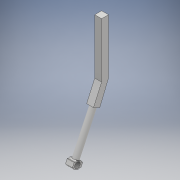
# Autodesk Inventor part: Fingers IPT
Saved by Autodesk Inventor 2017 (Build 210142000, 142)
## iProperties
Created: 2019-11-11
Part Number: Fingers IPT
Material: Generic
Document SubType Name: Modeling
Designer: kenli
Density: 1 g/cm^3
Appearance: Default
Author: kenli
Autodesk Inventor part; units mm, degrees
ref_plane "YZ Plane" through (0, 0, 0) normal (1, 0, 0) x (0, 1, 0)
ref_plane "XZ Plane" through (0, 0, 0) normal (0, 1, 0) x (-1, 0, 0)
ref_plane "XY Plane" through (0, 0, 0) normal (0, 0, 1) x (1, 0, 0)
sketch "Sketch1" plane through (0, 0, 0) normal (1, 0, 0) x (0, 1, 0)
  line L0 (3.4615, 28.4615) -> (-1.5385, 28.4615)
  line L1 (-1.5385, 28.4615) -> (-1.5385, -11.5385)
  line L2 (-1.5385, -11.5385) -> (3.4615, -11.5385)
  line L3 (3.4615, -11.5385) -> (3.4615, 28.4615)
  line L4 (3.4615, -11.5385) -> (-2.6923, -26.4744)
  line L5 (-2.8588, -26.8784) -> (-2.8558, -26.8796)
  line L6 (-2.8558, -26.8796) -> (-2.6923, -26.4744)
  line L7 (-2.8558, -26.8796) -> (-7.4503, -24.7123)
  line L8 (-7.4503, -24.7123) -> (-1.5385, -11.5385)
  point P0 (0, 0)
  dimension "d0" = 5
  dimension "d1" = 5.08
  dimension "d21" = 40
  constraints: 18 end point, 2 parallel, 2 perpendicular, 1 horizontal, 1 point on line
  measures "d0" distance between parallel lines of L1 L3
  measures "d1" distance of L5.end L7.end
  measures "d21" distance of L2.end L0.start
extrude "Extrusion1" add sketch "Sketch1" along normal blind 5
sketch "Sketch2" plane through (5, -2.8558, -26.8796) normal (0, -0.426635, -0.9044239) x (-1, 0, 0)
  circle A0 centre (2.5, -2.5) radius 2.0828
  line L0 (5, -5.08) -> (5, 0) projected
  line L1 (5, 0) -> (0, 0) projected
  point P0 (5, -8.885)
  dimension "d4" = 4.1656
  dimension "d5" = 2.5
  dimension "d6" = 2.5
  constraints: 1 centre point
  measures "d4" diameter of A0
  measures "d5" distance from line of A0.centre L0
  measures "d6" distance from line of A0.centre L1
extrude "Extrusion2" add sketch "Sketch2" along normal blind 30
sketch "Sketch7" plane through (2.5, -17.9159, -52.9458) normal (0, -0.426635, -0.9044239) x (-1, 0, 0)
  line L0 (2.5, -2.58) -> (-2.5, -2.58) projected
  line L1 (-2.5, 2.2849) -> (2.5, 2.2849)
  line L2 (2.5, 2.2849) -> (2.5, -2.58)
  line L3 (2.5, -2.58) -> (-2.5, -2.58)
  line L4 (-2.5, -2.58) -> (-2.5, 2.2849)
  point P0 (2.5, -6.385)
  constraints: 8 end point, 2 parallel, 1 horizontal, 1 perpendicular
extrude "Extrusion3" add sketch "Sketch7" along normal blind 5
sketch "Sketch8" plane through (0, -20.2493, -51.8451) normal (-1, 0, 0) x (0, 0.426635, 0.9044239)
  circle A0 centre (-2.5, 2.3649) radius 2.0828
  line L0 (-5, 0) -> (-5, 4.8649) projected
  line L1 (0, 4.8649) -> (-5, 4.8649) projected
  point P0 (55.529, -3.805)
  dimension "d13" = 4.1656
  dimension "d14" = 2.5
  dimension "d15" = 2.5
  constraints: 1 centre point
  measures "d13" diameter of A0
  measures "d14" distance from line of L0 A0.centre
  measures "d15" distance from line of A0.centre L1
extrude "Extrusion4" cut sketch "Sketch8" against normal blind 15
thread "Thread1" size "8-32 UNC" class "2B" standard "ANSI Unified Screw Threads" full length
fillet "Fillet1" radius 1 4 edges at (2.5, -22.3825, -56.3672) (2.5, -17.9826, -58.4427) (2.5, -15.8494, -53.9206) (2.5, -20.2493, -51.8451)
sketch "Sketch9" plane through (0, -20.6759, -52.7495) normal (0, -0.9044239, 0.426635) x (1, 0, 0)
  line L0 (0, -3.5828) -> (0, 0.5828) projected
  line L1 (5, 0) -> (5, -3) projected
  line L2 (0, 0.004) -> (5, 0.004)
  line L3 (5, 0.004) -> (5, -3)
  line L4 (5, -3) -> (0, -3)
  line L5 (0, -3) -> (0, 0.004)
  point P0 (0, 56.529)
  constraints: 8 end point, 2 parallel, 1 horizontal, 1 perpendicular, 1 point on line
extrude "Extrusion5" add sketch "Sketch9" along normal blind 1
sketch "Sketch10" plane through (0, -16.276, -54.825) normal (0, 0.9044239, -0.426635) x (1, 0, 0)
  point P0 (0, -56.529)
sketch "Sketch11" plane through (0, -16.276, -54.825) normal (0, 0.9044239, -0.426635) x (1, 0, 0)
  line L0 (5, -0.004) -> (5, -1) projected
  line L1 (0, 0) -> (0, 3) projected
  line L2 (5, -0.004) -> (0, -0.004)
  line L3 (0, -0.004) -> (0, 3)
  line L4 (0, 3) -> (5, 3)
  line L5 (5, 3) -> (5, -0.004)
  point P0 (0, -56.529)
  constraints: 8 end point, 2 parallel, 1 perpendicular
extrude "Extrusion6" add sketch "Sketch11" along normal blind 1
body "Solid1"
